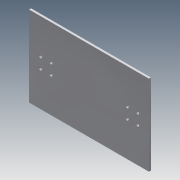
# Autodesk Inventor part: Y_CARRIAGE
Saved by Autodesk Inventor 2016 (Build 200138000, 138)
## iProperties
Created: 2017-05-10
Part Number: Y_CARRIAGE
Material: Generic
Document SubType Name: Modeling
Designer: Spark Electronics
Density: 1 g/cm^3
Appearance: Aluminum - Flat
Author: Spark Electronics
Autodesk Inventor part; units mm, degrees
ref_plane "YZ Plane" through (0, 0, 0) normal (1, 0, 0) x (0, 1, 0)
ref_plane "XZ Plane" through (0, 0, 0) normal (0, 1, 0) x (-1, 0, 0)
sketch "Sketch1" plane through (0, 0, 0) normal (0, 0, 1) x (1, 0, 0)
  line L0 (148, -99.5) -> (-148, -99.5)
  line L1 (-148, -99.5) -> (-148, 99.5)
  line L2 (-148, 99.5) -> (148, 99.5)
  line L3 (148, 99.5) -> (148, -99.5)
  line L4 (148, -99.5) -> (-148, 99.5) construction
  line L5 (-148, -99.5) -> (148, 99.5) construction
  circle A0 centre (-125.8625, 13) radius 2.5
  circle A1 centre (-125.8625, -13) radius 2.5
  circle A2 centre (-99.8625, 13) radius 2.5
  circle A3 centre (-99.8625, -13) radius 2.5
  line L6 (-125.8625, 13) -> (-125.8625, -13)
  line L7 (-125.8625, 0) -> (-98, 0)
  line L8 (0, 99.5) -> (0, -99.5) construction
  line L9 (-148, 0) -> (148, 0) construction
  circle A4 centre (125.8625, 13) radius 2.5
  circle A5 centre (125.8625, -13) radius 2.5
  circle A6 centre (99.8625, 13) radius 2.5
  circle A7 centre (99.8625, -13) radius 2.5
  line L10 (125.8625, 13) -> (125.8625, -13)
  line L11 (125.8625, 0) -> (98, 0)
  line L12 (148, 0) -> (-148, 0) construction
  point P0 (0, 0)
  dimension "d0" = 296
  dimension "d1" = 199
  dimension "d4" = 26
  dimension "d7" = 26
  dimension "d10" = 22.1375
  dimension "d14" = 5
  constraints: 26 end point, 8 centre point, 8 symmetric about line, 7 midpoint, 3 horizontal, 2 parallel, 2 vertical, 1 collinear, 1 perpendicular, 10 other
  measures "d0" distance of L1.end L2.end
  measures "d1" distance of L0.end L1.end
  measures "d4" distance of L6.start L6.end
  measures "d7" distance of L6.start A2.centre
  measures "d10" distance from line of L1 L6.start
  measures "d14" diameter of A0
extrude "Extrusion1" add sketch "Sketch1" along normal blind 5
hole "Hole1" at (-125.8625, 13, 5) direction (0, 0, -1) diameter 4.5 end through all countersink diameter 8 countersink angle 90
pattern_linear "Rectangular Pattern1" count 2 spacing 26 along (0, -1, 0) count 2 spacing 26 along (1, 0, 0) of "Hole1"
ref_plane "Work Plane1" through (0, -99.5, 0) normal (1, 0, 0) x (0, 0, -1)
mirror "Mirror1" about plane through (0, -99.5, 0) normal (1, 0, 0) of "Hole1", "Rectangular Pattern1"
body "Solid1"
